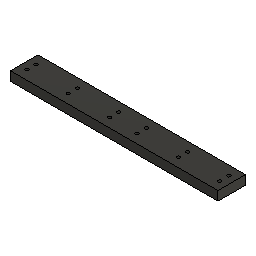
bar (Autodesk Fusion 360 design; units mm, degrees)
Autodesk Fusion 360 part; units mm, degrees
sketch "Skizze1" plane through (0, 0, 0) normal (0, 0, 1) x (1, 0, 0)
  line L0 (-127.7175, 0) -> (128.4747, 0) construction
  line L1 (0, 28.1433) -> (0, -31.677) construction
  line L2 (112.917, -15) -> (-112.917, -15)
  line L3 (-112.917, -15) -> (-112.917, 15)
  line L4 (-112.917, 15) -> (112.917, 15)
  line L5 (112.917, 15) -> (112.917, -15)
  line L6 (112.917, -15) -> (-112.917, 15) construction
  line L7 (-112.917, -15) -> (112.917, 15) construction
  line L8 (-118.6623, 5) -> (123.5472, 5) construction
  line L9 (-118.6623, -5) -> (120, -5) construction
  line L10 (15, 23.5796) -> (15, -25.7429) construction
  line L11 (-15, 27) -> (-15, -27) construction
  circle A0 centre (-15, 5) radius 1.75
  circle A1 centre (-15, -5) radius 1.75
  circle A2 centre (15, 5) radius 1.75
  circle A3 centre (15, -5) radius 1.75
  line L12 (-13.3257, 2.1) -> (-11.6514, 5)
  line L13 (-11.6514, 5) -> (-13.3257, 7.9)
  line L14 (-13.3257, 7.9) -> (-16.6743, 7.9)
  line L15 (-16.6743, 7.9) -> (-18.3486, 5)
  line L16 (-18.3486, 5) -> (-16.6743, 2.1)
  line L17 (-16.6743, 2.1) -> (-13.3257, 2.1)
  line L18 (-13.3257, -7.9) -> (-11.6514, -5)
  line L19 (-11.6514, -5) -> (-13.3257, -2.1)
  line L20 (-13.3257, -2.1) -> (-16.6743, -2.1)
  line L21 (-16.6743, -2.1) -> (-18.3486, -5)
  line L22 (-18.3486, -5) -> (-16.6743, -7.9)
  line L23 (-16.6743, -7.9) -> (-13.3257, -7.9)
  line L24 (16.6743, 2.1) -> (18.3486, 5)
  line L25 (18.3486, 5) -> (16.6743, 7.9)
  line L26 (16.6743, 7.9) -> (13.3257, 7.9)
  line L27 (13.3257, 7.9) -> (11.6514, 5)
  line L28 (11.6514, 5) -> (13.3257, 2.1)
  line L29 (13.3257, 2.1) -> (16.6743, 2.1)
  line L30 (16.6743, -7.9) -> (18.3486, -5)
  line L31 (18.3486, -5) -> (16.6743, -2.1)
  line L32 (16.6743, -2.1) -> (13.3257, -2.1)
  line L33 (13.3257, -2.1) -> (11.6514, -5)
  line L34 (11.6514, -5) -> (13.3257, -7.9)
  line L35 (13.3257, -7.9) -> (16.6743, -7.9)
  line L36 (58.3257, 7.9) -> (56.6514, 5)
  line L37 (56.6514, 5) -> (58.3257, 2.1)
  line L38 (58.3257, 2.1) -> (61.6743, 2.1)
  line L39 (61.6743, 2.1) -> (63.3486, 5)
  line L40 (63.3486, 5) -> (61.6743, 7.9)
  line L41 (61.6743, 7.9) -> (58.3257, 7.9)
  circle A4 centre (60, 5) radius 1.75
  line L42 (58.3257, -2.1) -> (56.6514, -5)
  line L43 (56.6514, -5) -> (58.3257, -7.9)
  line L44 (58.3257, -7.9) -> (61.6743, -7.9)
  line L45 (61.6743, -7.9) -> (63.3486, -5)
  line L46 (61.6743, -2.1) -> (58.3257, -2.1)
  line L47 (63.3486, -5) -> (61.6743, -2.1)
  circle A5 centre (60, -5) radius 1.75
  line L48 (103.3257, 7.9) -> (101.6514, 5)
  line L49 (101.6514, 5) -> (103.3257, 2.1)
  line L50 (103.3257, 2.1) -> (106.6743, 2.1)
  line L51 (106.6743, 2.1) -> (108.3486, 5)
  line L52 (108.3486, 5) -> (106.6743, 7.9)
  line L53 (106.6743, 7.9) -> (103.3257, 7.9)
  circle A6 centre (105, 5) radius 1.75
  line L54 (103.3257, -2.1) -> (101.6514, -5)
  line L55 (101.6514, -5) -> (103.3257, -7.9)
  line L56 (103.3257, -7.9) -> (106.6743, -7.9)
  line L57 (106.6743, -7.9) -> (108.3486, -5)
  line L58 (106.6743, -2.1) -> (103.3257, -2.1)
  line L59 (108.3486, -5) -> (106.6743, -2.1)
  circle A7 centre (105, -5) radius 1.75
  line L60 (-58.3257, 7.9) -> (-61.6743, 7.9)
  line L61 (-61.6743, 7.9) -> (-63.3486, 5)
  line L62 (-63.3486, 5) -> (-61.6743, 2.1)
  line L63 (-61.6743, 2.1) -> (-58.3257, 2.1)
  line L64 (-58.3257, 2.1) -> (-56.6514, 5)
  line L65 (-56.6514, 5) -> (-58.3257, 7.9)
  circle A8 centre (-60, 5) radius 1.75
  line L66 (-61.6743, -2.1) -> (-63.3486, -5)
  line L67 (-63.3486, -5) -> (-61.6743, -7.9)
  line L68 (-61.6743, -7.9) -> (-58.3257, -7.9)
  line L69 (-58.3257, -7.9) -> (-56.6514, -5)
  line L70 (-58.3257, -2.1) -> (-61.6743, -2.1)
  line L71 (-56.6514, -5) -> (-58.3257, -2.1)
  circle A9 centre (-60, -5) radius 1.75
  line L72 (-103.3257, 7.9) -> (-106.6743, 7.9)
  line L73 (-106.6743, 7.9) -> (-108.3486, 5)
  line L74 (-108.3486, 5) -> (-106.6743, 2.1)
  line L75 (-106.6743, 2.1) -> (-103.3257, 2.1)
  line L76 (-103.3257, 2.1) -> (-101.6514, 5)
  line L77 (-101.6514, 5) -> (-103.3257, 7.9)
  circle A10 centre (-105, 5) radius 1.75
  line L78 (-106.6743, -2.1) -> (-108.3486, -5)
  line L79 (-108.3486, -5) -> (-106.6743, -7.9)
  line L80 (-106.6743, -7.9) -> (-103.3257, -7.9)
  line L81 (-103.3257, -7.9) -> (-101.6514, -5)
  line L82 (-103.3257, -2.1) -> (-106.6743, -2.1)
  line L83 (-101.6514, -5) -> (-103.3257, -2.1)
  circle A11 centre (-105, -5) radius 1.75
  point P0 (-15, 5)
  point P1 (-15, -5)
  point P2 (15, 5)
  point P3 (15, -5)
  dimension "d1" = 225.834
  dimension "d2" = 30
  dimension "d3" = 5
  dimension "d4" = 5
  dimension "d5" = 15
  dimension "d6" = 15
  dimension "d7" = 3.5
  dimension "d8" = 3.5
  dimension "d9" = 3.5
  dimension "d10" = 3.5
  dimension "d11" = 5.8
  dimension "d12" = 5.8
  dimension "d13" = 5.8
  dimension "d14" = 5.8
  dimension "d17" = 90
  dimension "d18" = 0
  dimension "d21" = -90
  dimension "d22" = 0
  constraint horizontal L0
  constraint coincident origin L0
  constraint perpendicular L0 L1
  constraint coincident origin L1
  constraint horizontal L2
  constraint perpendicular L2 L3
  constraint parallel L2 L4
  constraint parallel L3 L5
  constraint coincident L6 origin
  constraint coincident L7 origin
  constraint perpendicular L5 L8
  constraint perpendicular L5 L9
  constraint perpendicular L2 L10
  constraint perpendicular L9 L11
  constraint coincident L8 P0
  constraint coincident L11 P0
  constraint coincident L9 P1
  constraint coincident L11 P1
  constraint coincident L8 P2
  constraint coincident L10 P2
  constraint coincident L9 P3
  constraint coincident L10 P3
  constraint coincident P0 A0.centre
  constraint coincident P1 A1.centre
  constraint coincident P2 A2.centre
  constraint coincident P3 A3.centre
  constraint horizontal L29
  constraint horizontal L35
  constraint horizontal L23
  constraint horizontal L17
  measures "d1" distance of L3 L5
  measures "d2" distance of L2 L4
  measures "d3" distance of L0 L8
  measures "d4" distance of L0 L9
  measures "d5" distance of L1 L10
  measures "d6" distance of L1 L11
  measures "d7" diameter of A2
  measures "d8" diameter of A3
  measures "d9" diameter of A0
  measures "d10" diameter of A1
  measures "d11" distance of L26 L29
  measures "d12" distance of L32 L35
  measures "d13" distance of L20 L23
  measures "d14" distance of L14 L17
extrude "Extrusion1" add sketch "Skizze1" along normal blind 10 contours L2 L3 L4 L5 | L12 L13 L14 L15 L16 L17 | L18 L19 L20 L21 L22 L23 | L24 L25 L26 L27 L28 L29 | L30 L31 L32 L33 L34 L35 | L36 L37 L38 L39 L40 L41 | L42 L43 L44 L45 L46 L47 | L48 L49 L50 L51 L52 L53 | L54 L55 L56 L57 L58 L59 | L60 L61 L62 L63 L64 L65 | L66 L67 L68 L69 L70 L71 | L72 L73 L74 L75 L76 L77 | L78 L79 L80 L81 L82 L83
extrude "Extrusion2" cut sketch "Skizze1" along normal blind 7 contours L12 L13 L14 L15 L16 L17 | L18 L19 L20 L21 L22 L23 | L24 L25 L26 L27 L28 L29 | L30 L31 L32 L33 L34 L35 | L36 L37 L38 L39 L40 L41 | L42 L43 L44 L45 L46 L47 | L48 L49 L50 L51 L52 L53 | L54 L55 L56 L57 L58 L59 | L60 L61 L62 L63 L64 L65 | L66 L67 L68 L69 L70 L71 | L72 L73 L74 L75 L76 L77 | L78 L79 L80 L81 L82 L83
extrude "Extrusion3" add sketch "Skizze1" along normal blind 4.3 contours L12 L13 L14 L15 L16 L17 | L18 L19 L20 L21 L22 L23 | L24 L25 L26 L27 L28 L29 | L30 L31 L32 L33 L34 L35 | L36 L37 L38 L39 L40 L41 | L42 L43 L44 L45 L46 L47 | L48 L49 L50 L51 L52 L53 | L54 L55 L56 L57 L58 L59 | L60 L61 L62 L63 L64 L65 | L66 L67 L68 L69 L70 L71 | L72 L73 L74 L75 L76 L77 | L78 L79 L80 L81 L82 L83
named bodies: "bar"
